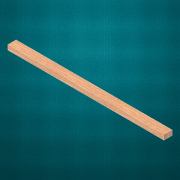
# Autodesk Inventor part: Suspension Brace
Saved by Autodesk Inventor 2017 (Build 210142000, 142)
## iProperties
Created: 2017-09-04
Part Number: Suspension Brace
Material: Wood (Birch)
Document SubType Name: Modeling
Designer: Michael
Density: 0.55 g/cm^3
Appearance: Birch - Natural Polished
Author: Michael
Autodesk Inventor part; units mm, degrees
ref_plane "YZ Plane" through (0, 0, 0) normal (1, 0, 0) x (0, 1, 0)
ref_plane "XZ Plane" through (0, 0, 0) normal (0, 1, 0) x (-1, 0, 0)
ref_plane "XY Plane" through (0, 0, 0) normal (0, 0, 1) x (1, 0, 0)
sketch "Sketch1" plane through (0, 0, 0) normal (1, 0, 0) x (0, 1, 0)
  line L0 (-11.1125, 19.05) -> (11.1125, 19.05)
  line L1 (11.1125, 19.05) -> (11.1125, -19.05)
  line L2 (11.1125, -19.05) -> (-11.1125, -19.05)
  line L3 (-11.1125, -19.05) -> (-11.1125, 19.05)
  line L4 (-11.1125, 19.05) -> (11.1125, -19.05) construction
  line L5 (11.1125, 19.05) -> (-11.1125, -19.05) construction
  point P0 (0, 0)
  dimension "d0" = 38.1
  dimension "d1" = 22.225
  constraints: 12 end point, 2 midpoint, 2 parallel, 1 horizontal, 1 perpendicular
  measures "d0" distance of L0.end L1.end
  measures "d1" distance of L0.start L0.end
extrude "Extrusion1" add sketch "Sketch1" along normal mid plane 717.55
body "Solid1"
